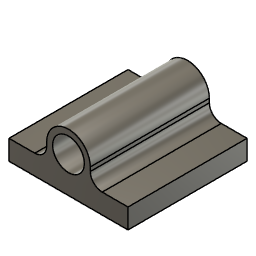
cable tie base (Autodesk Fusion 360 design; units mm, degrees)
Autodesk Fusion 360 part; units mm, degrees
sketch "Sketch1" plane through (0, 0, 0) normal (0, 1, 0) x (1, 0, 0)
  line L0 (-40.1743, 28.9794) -> (-10.1743, 28.9794)
  line L1 (-10.1743, 28.9794) -> (-10.1743, -1.0206)
  line L2 (-10.1743, -1.0206) -> (-40.1743, -1.0206)
  line L3 (-40.1743, -1.0206) -> (-40.1743, 28.9794)
  dimension "d1" = 30
  dimension "d2" = 30
  constraint horizontal L0
  constraint vertical L1
  constraint horizontal L2
  constraint vertical L3
  measures "d1" distance of L0.start L0.end
  measures "d2" distance of L0.start L2.end
extrude "Extrude1" add sketch "Sketch1" along normal blind 5
sketch "Sketch2" plane through (0, 0, 1.0206) normal (0, 0, 1) x (1, 0, 0)
  line L0 (-40.1743, 0) -> (-10.1743, 0)
  line L1 (-10.1743, 0) -> (-10.1743, 5)
  line L2 (-10.1743, 5) -> (-40.1743, 5)
  line L3 (-40.1743, 5) -> (-40.1743, 0)
  circle A0 centre (-25.1743, 9) radius 4
  circle A1 centre (-25.1743, 9) radius 5.5
  line L4 (-19.6743, 9) -> (-19.6743, 5)
  line L5 (-30.6743, 9) -> (-30.6743, 4.9999)
  dimension "d8" = 8
  dimension "d9" = 11
  constraint coincident A1 L5.start
  constraint coincident A1 L4.start
  constraint coincident L2 L4.end
  constraint tangent A1 L4
  constraint vertical L5
  measures "d8" diameter of A0
  measures "d9" diameter of A1
extrude "Extrude2" add sketch "Sketch2" against normal blind 30 contours L2 A1 L5 | L2 A1 L4 | L2 A1 picked at (-30.1523, 9.3387)
fillet "Fillet1" radius 3 2 edges at (-19.6743, 5, -13.9794) (-30.6743, 5, -13.9794)
